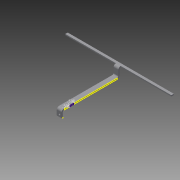
# Autodesk Inventor part: Feeder-Grabber_v1
Saved by Autodesk Inventor 2013 (Build 170138000, 138)
## iProperties
Created: 2013-01-21
Part Number: Feeder-Grabber_v1
Material: Generic
Document SubType Name: Sheet Metal
Designer: motoennies
Density: 1 g/cm^3
Sheet Metal Rule: Default
Author: motoennies
Autodesk Inventor part; units mm, degrees
ref_plane "YZ Plane" through (0, 0, 0) normal (1, 0, 0) x (0, 1, 0)
ref_plane "XZ Plane" through (0, 0, 0) normal (0, 1, 0) x (-1, 0, 0)
ref_plane "XY Plane" through (0, 0, 0) normal (0, 0, 1) x (1, 0, 0)
sketch "Sketch1" plane through (0, 0, 0) normal (0, 0, 1) x (1, 0, 0)
  line L0 (0, 0) -> (-12.7, 0)
  line L1 (-12.7, 0) -> (-12.7, 19.05)
  line L2 (-12.7, 19.05) -> (0, 19.05)
  line L3 (0, 19.05) -> (0, 0)
  dimension "d0" = 12.7
  dimension "d1" = 19.05
  measures "d0" distance of L0.start L0.end
  measures "d1" distance of L0.end L1.end
extrude "Plate1" add sketch "Sketch1" along normal blind 3.048
sketch "Sketch2" plane through (0, 16.002, 3.048) normal (0, 1, 0) x (-1, 0, 0)
  line L0 (12.7, 0) -> (0, 0)
  line L1 (0, 0) -> (0, -152.4)
  line L2 (0, -152.4) -> (12.7, -152.4)
  line L3 (12.7, -152.4) -> (12.7, 0)
  constraints: 6 end point, 1 horizontal, 1 perpendicular, 1 vertical
edge flange "Flange1" height 152.4 angle 90 thickness 3.048 bend radius 3.175 thickness toward (0, 1, 0) relief straight relief width 3.048 relief depth 1.524 edges at (-6.35, 19.05, 0) wall of the first edge with corners at (-12.7, 16.002, 3.048) (0, 16.002, 3.048) (0, 16.002, -149.352) (-12.7, 16.002, -149.352)
bend "Bend1"
corner "Corner1"
sketch "Sketch3" plane through (0, 0, 3.048) normal (0, 0, 1) x (1, 0, 0)
  line L0 (0, 12.827) -> (-12.7, 12.827) projected
  line L1 (0, 12.827) -> (0, 0) projected
  circle A0 centre (-6.35, 6.4135) radius 2.54
  dimension "d13" = 5.08
  dimension "d15" = 6.4135
  dimension "d16" = 6.35
  constraints: 1 centre point
  measures "d13" diameter of A0
  measures "d15" distance from line of L0 A0.centre
  measures "d16" distance from line of L1 A0.centre
extrude "Cut1" cut sketch "Sketch3" against normal blind 3.048
sketch "Sketch4" plane through (-12.7, 16.002, -146.304) normal (0, 0, -1) x (-1, 0, 0)
  line L0 (-12.7, 0) -> (0, 0)
  line L1 (0, 0) -> (0, 25.4)
  line L2 (0, 25.4) -> (-12.7, 25.4)
  line L3 (-12.7, 25.4) -> (-12.7, 0)
  constraints: 6 end point, 1 horizontal, 1 perpendicular, 1 vertical
edge flange "Flange2" height 25.4 angle 90 thickness 3.048 bend radius 3.175 thickness toward (0, 0, -1) relief straight relief width 3.048 relief depth 1.524 edges at (-6.35, 19.05, -149.352) wall of the first edge with corners at (0, 16.002, -146.304) (-12.7, 16.002, -146.304) (-12.7, 41.402, -146.304) (0, 41.402, -146.304)
bend "Bend2"
corner "Corner2"
sketch "Sketch5" plane through (0, 38.354, -146.304) normal (0, 1, 0) x (-1, 0, 0)
  line L0 (12.7, 0) -> (0, 0)
  line L1 (0, 0) -> (0, -12.7)
  line L2 (0, -12.7) -> (12.7, -12.7)
  line L3 (12.7, -12.7) -> (12.7, 0)
  constraints: 6 end point, 1 horizontal, 1 perpendicular, 1 vertical
edge flange "Flange3" height 12.7 angle 90 thickness 3.048 bend radius 3.175 thickness toward (0, 1, 0) relief straight relief width 3.048 relief depth 1.524 edges at (-6.35, 41.402, -149.352) wall of the first edge with corners at (-12.7, 38.354, -146.304) (0, 38.354, -146.304) (0, 38.354, -159.004) (-12.7, 38.354, -159.004)
bend "Bend3"
corner "Corner3"
sketch "Sketch6" plane through (0, 38.354, -159.004) normal (1, 0, 0) x (0, 0, -1)
  line L0 (-6.477, 3.048) -> (-6.477, 0) projected
  line L1 (0, 0) -> (-6.477, 0) projected
  line L2 (0, 0) -> (0, 3.048) projected
  line L3 (0, 3.048) -> (-6.477, 3.048) projected
  point P0 (-159.004, -38.354)
extrude "Extrusion1" add sketch "Sketch6" along normal blind 133.35
sketch "Sketch7" plane through (-12.7, 38.354, -159.004) normal (-1, 0, 0) x (0, 0, 1)
  line L0 (6.477, 0) -> (6.477, 3.048) projected
  line L1 (6.477, 3.048) -> (0, 3.048) projected
  line L2 (0, 0) -> (0, 3.048) projected
  line L3 (0, 0) -> (6.477, 0) projected
  point P0 (159.004, -38.354)
extrude "Extrusion2" add sketch "Sketch7" along normal blind 133.35
sketch "Sketch8" plane through (0, 16.002, -3.175) normal (1, 0, 0) x (0, 0, -1)
  line L0 (139.954, 0) -> (139.954, 3.048) projected
  line L1 (139.954, 3.048) -> (0, 3.048) projected
  line L2 (0, 3.048) -> (0, 0) projected
  line L3 (139.954, 0) -> (0, 0) projected
  line L4 (12.7, 3.048) -> (25.4, 3.048)
  line L5 (25.4, 3.048) -> (25.4, 0)
  line L6 (25.4, 0) -> (12.7, 0)
  line L7 (12.7, 3.048) -> (12.7, 0)
  point P0 (-3.175, -16.002)
  dimension "d43" = 12.7
  dimension "d44" = 12.7
  constraints: 8 end point, 4 point on line, 2 perpendicular
  measures "d43" distance of L4.start L4.end
  measures "d44" distance between parallel lines of L2 L7
equation "\"d17\" = Thickness"
equation "\"d3\" = BendReliefWidth"
equation "\"d4\" = BendReliefDepth"
equation "\"d5\" = MinimumRemnant"
equation "\"d6\" = BendRadius"
equation "\"d10\" = CornerReliefSize"
equation "\"d11\" = GapSize"
equation "\"d12\" = JacobiRadiusSize"
equation "\"d19\" = BendReliefWidth"
equation "\"d20\" = BendReliefDepth"
equation "\"d21\" = MinimumRemnant"
equation "\"d22\" = BendRadius"
equation "\"d26\" = CornerReliefSize"
equation "\"d27\" = GapSize"
equation "\"d28\" = JacobiRadiusSize"
equation "\"d29\" = BendReliefWidth"
equation "\"d30\" = BendReliefDepth"
equation "\"d31\" = MinimumRemnant"
equation "\"d32\" = BendRadius"
equation "\"d36\" = CornerReliefSize"
equation "\"d37\" = GapSize"
equation "\"d38\" = JacobiRadiusSize"
equation "\"BendRadius\" = Thickness"
equation "\"BendReliefWidth\" = Thickness"
equation "\"BendReliefDepth\" = 0.5 * Thickness"
equation "\"CornerReliefSize\" = 4 * Thickness"
equation "\"MinimumRemnant\" = 2 * Thickness"
equation "\"TransitionRadius\" = BendRadius"
equation "\"JacobiRadiusSize\" = BendRadius"
equation "\"GapSize\" = Thickness"
equation "\"d2\" = BendRadius"
equation "\"Thickness\" = 3.048"
body "Solid1"
